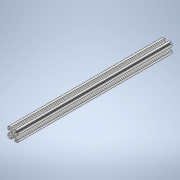
# Autodesk Inventor part: TurretSupp2
Saved by Autodesk Inventor 2022 (Build 260153000, 153)
## iProperties
Created: 2022-01-17
Part Number: TurretSupp2
Material: Generic
Document SubType Name: Modeling
Designer: Ty Gazaway
Density: 1 g/cm^3
Appearance: Default
Author: Ty Gazaway
Autodesk Inventor part; units mm, degrees
ref_plane "YZ Plane" through (0, 0, 0) normal (1, 0, 0) x (0, 1, 0)
ref_plane "XZ Plane" through (0, 0, 0) normal (0, 1, 0) x (-1, 0, 0)
ref_plane "Work Plane1" through (4.7107, 12.7, 500) normal (0, 0, 1) x (1, 0, 0)
sketch "Sketch1" plane through (4.7107, 12.7, 500) normal (0, 0, 1) x (1, 0, 0)
  line L0 (2.275, -4.583) -> (2.7779, -4.0801) projected
  arc A0 (2.7779, -4.0801) -> (2.8386, -3.8252) centre (2.6011, -3.9033) ccw projected
  arc A1 (5.1826, -1.1279) -> (2.8386, -3.8252) centre (4.8143, -3.175) ccw projected
  arc A2 (5.1826, -1.1279) -> (5.7159, -0.4073) centre (5.2712, -0.6358) ccw projected
  arc A3 (5.7159, -0.4073) -> (5.0488, 0) centre (5.0488, -0.75) ccw projected
  line L1 (5.0488, 0) -> (0, 0) projected
  arc A4 (0, 0) -> (-0.5303, -0.2197) centre (0, -0.75) ccw projected
  line L2 (-0.5303, -0.2197) -> (-1.7399, -1.4293) projected
  arc A5 (-1.7399, -1.4293) -> (-1.6692, -1.6) centre (-1.6692, -1.5) ccw projected
  line L3 (-1.6692, -1.6) -> (-0.3857, -1.6) projected
  arc A6 (0.1143, -2.1) -> (-0.3857, -1.6) centre (-0.3857, -2.1) ccw projected
  line L4 (0.1143, -2.1) -> (0.1143, -6.1) projected
  arc A7 (-1.3857, -7.6) -> (0.1143, -6.1) centre (-1.3857, -6.1) ccw projected
  line L5 (-1.3857, -7.6) -> (-1.5607, -7.6) projected
  arc A8 (-1.5607, -7.6) -> (-2.0607, -8.1) centre (-1.5607, -8.1) ccw projected
  arc A9 (-3.0607, -9.1) -> (-2.0607, -8.1) centre (-3.0607, -8.1) ccw projected
  line L6 (-3.0607, -9.1) -> (-6.3607, -9.1) projected
  arc A10 (-7.3607, -8.1) -> (-6.3607, -9.1) centre (-6.3607, -8.1) ccw projected
  arc A11 (-7.3607, -8.1) -> (-7.8607, -7.6) centre (-7.8607, -8.1) ccw projected
  line L7 (-7.8607, -7.6) -> (-8.0357, -7.6) projected
  arc A12 (-9.5357, -6.1) -> (-8.0357, -7.6) centre (-8.0357, -6.1) ccw projected
  line L8 (-9.5357, -6.1) -> (-9.5357, -2.1) projected
  arc A13 (-9.0357, -1.6) -> (-9.5357, -2.1) centre (-9.0357, -2.1) ccw projected
  line L9 (-9.0357, -1.6) -> (-7.7521, -1.6) projected
  arc A14 (-7.7521, -1.6) -> (-7.6814, -1.4293) centre (-7.7521, -1.5) ccw projected
  line L10 (-7.6814, -1.4293) -> (-8.891, -0.2197) projected
  arc A15 (-8.891, -0.2197) -> (-9.4213, 0) centre (-9.4213, -0.75) ccw projected
  line L11 (-9.4213, 0) -> (-14.4701, 0) projected
  arc A16 (-14.4701, 0) -> (-15.1372, -0.4073) centre (-14.4701, -0.75) ccw projected
  arc A17 (-15.1372, -0.4073) -> (-14.6039, -1.1279) centre (-14.6925, -0.6358) ccw projected
  arc A18 (-12.2599, -3.8252) -> (-14.6039, -1.1279) centre (-14.2357, -3.175) ccw projected
  arc A19 (-12.2599, -3.8252) -> (-12.1992, -4.0801) centre (-12.0224, -3.9033) ccw projected
  line L12 (-12.1992, -4.0801) -> (-11.6963, -4.583) projected
  arc A20 (-11.6963, -5.2901) -> (-11.6963, -4.583) centre (-12.0499, -4.9365) ccw projected
  line L13 (-11.6963, -5.2901) -> (-12.1206, -5.7144) projected
  arc A21 (-12.8277, -5.7144) -> (-12.1206, -5.7144) centre (-12.4741, -5.3608) ccw projected
  line L14 (-12.8277, -5.7144) -> (-13.3306, -5.2115) projected
  arc A22 (-13.3306, -5.2115) -> (-13.5855, -5.1508) centre (-13.5073, -5.3882) ccw projected
  arc A23 (-16.2828, -2.8067) -> (-13.5855, -5.1508) centre (-14.2357, -3.175) ccw projected
  arc A24 (-16.2828, -2.8067) -> (-17.0034, -2.2734) centre (-16.7749, -2.7182) ccw projected
  arc A25 (-17.0034, -2.2734) -> (-17.4107, -2.9406) centre (-16.6607, -2.9406) ccw projected
  line L15 (-17.4107, -2.9406) -> (-17.4107, -7.9893) projected
  arc A26 (-17.4107, -7.9893) -> (-17.191, -8.5197) centre (-16.6607, -7.9893) ccw projected
  line L16 (-17.191, -8.5197) -> (-15.9814, -9.7293) projected
  arc A27 (-15.9814, -9.7293) -> (-15.8107, -9.6586) centre (-15.9107, -9.6586) ccw projected
  line L17 (-15.8107, -9.6586) -> (-15.8107, -8.375) projected
  arc A28 (-15.3107, -7.875) -> (-15.8107, -8.375) centre (-15.3107, -8.375) ccw projected
  line L18 (-15.3107, -7.875) -> (-11.3107, -7.875) projected
  arc A29 (-9.8107, -9.375) -> (-11.3107, -7.875) centre (-11.3107, -9.375) ccw projected
  line L19 (-9.8107, -9.375) -> (-9.8107, -9.55) projected
  arc A30 (-9.8107, -9.55) -> (-9.3107, -10.05) centre (-9.3107, -9.55) ccw projected
  arc A31 (-8.3107, -11.05) -> (-9.3107, -10.05) centre (-9.3107, -11.05) ccw projected
  line L20 (-8.3107, -11.05) -> (-8.3107, -14.35) projected
  arc A32 (-9.3107, -15.35) -> (-8.3107, -14.35) centre (-9.3107, -14.35) ccw projected
  arc A33 (-9.3107, -15.35) -> (-9.8107, -15.85) centre (-9.3107, -15.85) ccw projected
  line L21 (-9.8107, -15.85) -> (-9.8107, -16.025) projected
  arc A34 (-11.3107, -17.525) -> (-9.8107, -16.025) centre (-11.3107, -16.025) ccw projected
  line L22 (-11.3107, -17.525) -> (-15.3107, -17.525) projected
  arc A35 (-15.8107, -17.025) -> (-15.3107, -17.525) centre (-15.3107, -17.025) ccw projected
  line L23 (-15.8107, -17.025) -> (-15.8107, -15.7414) projected
  arc A36 (-15.8107, -15.7414) -> (-15.9814, -15.6707) centre (-15.9107, -15.7414) ccw projected
  line L24 (-15.9814, -15.6707) -> (-17.191, -16.8803) projected
  arc A37 (-17.191, -16.8803) -> (-17.4107, -17.4107) centre (-16.6607, -17.4107) ccw projected
  line L25 (-17.4107, -17.4107) -> (-17.4107, -22.4594) projected
  arc A38 (-17.4107, -22.4594) -> (-17.0034, -23.1266) centre (-16.6607, -22.4594) ccw projected
  arc A39 (-17.0034, -23.1266) -> (-16.2828, -22.5933) centre (-16.7749, -22.6818) ccw projected
  arc A40 (-13.5855, -20.2492) -> (-16.2828, -22.5933) centre (-14.2357, -22.225) ccw projected
  arc A41 (-13.5855, -20.2492) -> (-13.3306, -20.1885) centre (-13.5073, -20.0118) ccw projected
  line L26 (-13.3306, -20.1885) -> (-12.8277, -19.6856) projected
  arc A42 (-12.1206, -19.6856) -> (-12.8277, -19.6856) centre (-12.4741, -20.0392) ccw projected
  line L27 (-12.1206, -19.6856) -> (-11.6963, -20.1099) projected
  arc A43 (-11.6963, -20.817) -> (-11.6963, -20.1099) centre (-12.0499, -20.4635) ccw projected
  line L28 (-11.6963, -20.817) -> (-12.1992, -21.3199) projected
  arc A44 (-12.1992, -21.3199) -> (-12.2599, -21.5748) centre (-12.0224, -21.4967) ccw projected
  arc A45 (-14.6039, -24.2721) -> (-12.2599, -21.5748) centre (-14.2357, -22.225) ccw projected
  arc A46 (-14.6039, -24.2721) -> (-15.1372, -24.9927) centre (-14.6925, -24.7642) ccw projected
  arc A47 (-15.1372, -24.9927) -> (-14.4701, -25.4) centre (-14.4701, -24.65) ccw projected
  line L29 (-14.4701, -25.4) -> (-9.4213, -25.4) projected
  arc A48 (-9.4213, -25.4) -> (-8.891, -25.1803) centre (-9.4213, -24.65) ccw projected
  line L30 (-8.891, -25.1803) -> (-7.6814, -23.9707) projected
  arc A49 (-7.6814, -23.9707) -> (-7.7521, -23.8) centre (-7.7521, -23.9) ccw projected
  line L31 (-7.7521, -23.8) -> (-9.0357, -23.8) projected
  arc A50 (-9.5357, -23.3) -> (-9.0357, -23.8) centre (-9.0357, -23.3) ccw projected
  line L32 (-9.5357, -23.3) -> (-9.5357, -19.3) projected
  arc A51 (-8.0357, -17.8) -> (-9.5357, -19.3) centre (-8.0357, -19.3) ccw projected
  line L33 (-8.0357, -17.8) -> (-7.8607, -17.8) projected
  arc A52 (-7.8607, -17.8) -> (-7.3607, -17.3) centre (-7.8607, -17.3) ccw projected
  arc A53 (-6.3607, -16.3) -> (-7.3607, -17.3) centre (-6.3607, -17.3) ccw projected
  line L34 (-6.3607, -16.3) -> (-3.0607, -16.3) projected
  arc A54 (-2.0607, -17.3) -> (-3.0607, -16.3) centre (-3.0607, -17.3) ccw projected
  arc A55 (-2.0607, -17.3) -> (-1.5607, -17.8) centre (-1.5607, -17.3) ccw projected
  line L35 (-1.5607, -17.8) -> (-1.3857, -17.8) projected
  arc A56 (0.1143, -19.3) -> (-1.3857, -17.8) centre (-1.3857, -19.3) ccw projected
  line L36 (0.1143, -19.3) -> (0.1143, -23.3) projected
  arc A57 (-0.3857, -23.8) -> (0.1143, -23.3) centre (-0.3857, -23.3) ccw projected
  line L37 (-0.3857, -23.8) -> (-1.6692, -23.8) projected
  arc A58 (-1.6692, -23.8) -> (-1.7399, -23.9707) centre (-1.6692, -23.9) ccw projected
  line L38 (-1.7399, -23.9707) -> (-0.5303, -25.1803) projected
  arc A59 (-0.5303, -25.1803) -> (0, -25.4) centre (0, -24.65) ccw projected
  line L39 (0, -25.4) -> (5.0488, -25.4) projected
  arc A60 (5.0488, -25.4) -> (5.7159, -24.9927) centre (5.0488, -24.65) ccw projected
  arc A61 (5.7159, -24.9927) -> (5.1826, -24.2721) centre (5.2712, -24.7642) ccw projected
  arc A62 (2.8386, -21.5748) -> (5.1826, -24.2721) centre (4.8143, -22.225) ccw projected
  arc A63 (2.8386, -21.5748) -> (2.7779, -21.3199) centre (2.6011, -21.4967) ccw projected
  line L40 (2.7779, -21.3199) -> (2.275, -20.817) projected
  arc A64 (2.275, -20.1099) -> (2.275, -20.817) centre (2.6285, -20.4635) ccw projected
  line L41 (2.275, -20.1099) -> (2.6992, -19.6856) projected
  arc A65 (3.4064, -19.6856) -> (2.6992, -19.6856) centre (3.0528, -20.0392) ccw projected
  line L42 (3.4064, -19.6856) -> (3.9092, -20.1885) projected
  arc A66 (3.9092, -20.1885) -> (4.1642, -20.2492) centre (4.086, -20.0118) ccw projected
  arc A67 (6.8615, -22.5933) -> (4.1642, -20.2492) centre (4.8143, -22.225) ccw projected
  arc A68 (6.8615, -22.5933) -> (7.582, -23.1266) centre (7.3536, -22.6818) ccw projected
  arc A69 (7.582, -23.1266) -> (7.9893, -22.4594) centre (7.2393, -22.4594) ccw projected
  line L43 (7.9893, -22.4594) -> (7.9893, -17.4107) projected
  arc A70 (7.9893, -17.4107) -> (7.7697, -16.8803) centre (7.2393, -17.4107) ccw projected
  line L44 (7.7697, -16.8803) -> (6.5601, -15.6707) projected
  arc A71 (6.5601, -15.6707) -> (6.3893, -15.7414) centre (6.4893, -15.7414) ccw projected
  line L45 (6.3893, -15.7414) -> (6.3893, -17.025) projected
  arc A72 (5.8893, -17.525) -> (6.3893, -17.025) centre (5.8893, -17.025) ccw projected
  line L46 (5.8893, -17.525) -> (1.8893, -17.525) projected
  arc A73 (0.3893, -16.025) -> (1.8893, -17.525) centre (1.8893, -16.025) ccw projected
  line L47 (0.3893, -16.025) -> (0.3893, -15.85) projected
  arc A74 (0.3893, -15.85) -> (-0.1107, -15.35) centre (-0.1107, -15.85) ccw projected
  arc A75 (-1.1107, -14.35) -> (-0.1107, -15.35) centre (-0.1107, -14.35) ccw projected
  line L48 (-1.1107, -14.35) -> (-1.1107, -11.05) projected
  arc A76 (-0.1107, -10.05) -> (-1.1107, -11.05) centre (-0.1107, -11.05) ccw projected
  arc A77 (-0.1107, -10.05) -> (0.3893, -9.55) centre (-0.1107, -9.55) ccw projected
  line L49 (0.3893, -9.55) -> (0.3893, -9.375) projected
  arc A78 (1.8893, -7.875) -> (0.3893, -9.375) centre (1.8893, -9.375) ccw projected
  line L50 (1.8893, -7.875) -> (5.8893, -7.875) projected
  arc A79 (6.3893, -8.375) -> (5.8893, -7.875) centre (5.8893, -8.375) ccw projected
  line L51 (6.3893, -8.375) -> (6.3893, -9.6586) projected
  arc A80 (6.3893, -9.6586) -> (6.5601, -9.7293) centre (6.4893, -9.6586) ccw projected
  line L52 (6.5601, -9.7293) -> (7.7697, -8.5197) projected
  arc A81 (7.7697, -8.5197) -> (7.9893, -7.9893) centre (7.2393, -7.9893) ccw projected
  line L53 (7.9893, -7.9893) -> (7.9893, -2.9406) projected
  arc A82 (7.9893, -2.9406) -> (7.582, -2.2734) centre (7.2393, -2.9406) ccw projected
  arc A83 (7.582, -2.2734) -> (6.8615, -2.8067) centre (7.3536, -2.7182) ccw projected
  arc A84 (4.1642, -5.1508) -> (6.8615, -2.8067) centre (4.8143, -3.175) ccw projected
  arc A85 (4.1642, -5.1508) -> (3.9092, -5.2115) centre (4.086, -5.3882) ccw projected
  line L54 (3.9092, -5.2115) -> (3.4064, -5.7144) projected
  arc A86 (2.6992, -5.7144) -> (3.4064, -5.7144) centre (3.0528, -5.3608) ccw projected
  line L55 (2.6992, -5.7144) -> (2.275, -5.2901) projected
  arc A87 (2.275, -4.583) -> (2.275, -5.2901) centre (2.6285, -4.9365) ccw projected
  circle A88 centre (-4.7107, -12.7) radius 2.08 projected
extrude "Extrusion1" add sketch "Sketch1" along normal blind 368.3
body "Solid1"
